# Autodesk Inventor part: LED1_CHIPLED_0805
Saved by Autodesk Inventor 2016 (Build 200138000, 138)
## iProperties
Created: 2016-04-08
Part Number: LED1_CHIPLED_0805
Material: Generic
Document SubType Name: Modeling
Designer: Paschalis
Density: 1 g/cm^3
Appearance: CHIPLED_0805, LED1_CHIPLED_0805
Author: Paschalis
Autodesk Inventor part; units mm, degrees
ref_plane "YZ Plane" through (0, 0, 0) normal (1, 0, 0) x (0, 1, 0)
ref_plane "XZ Plane" through (0, 0, 0) normal (0, 1, 0) x (-1, 0, 0)
ref_plane "XY Plane" through (0, 0, 0) normal (0, 0, 1) x (1, 0, 0)
sketch "CHIPLED_0805, LED1_CHIPLED_0805_77" plane through (0, 0, 0) normal (0, 0, 1) x (1, 0, 0)
  line L0 (-0.625, 1.0508) -> (0.625, 1.0508)
  line L1 (0.625, 1.0508) -> (0.625, -1)
  line L2 (0.625, -1) -> (-0.625, -1)
  line L3 (-0.625, -1) -> (-0.625, 1.0508)
  constraints: 8 end point
extrude "Extrusion1" add sketch "CHIPLED_0805, LED1_CHIPLED_0805_77" along normal blind 1
body "Solid1"
